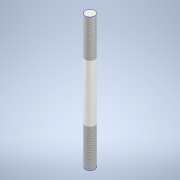
# Autodesk Inventor part: M5_60_shaft
Saved by Autodesk Inventor 2020.3 (Build 243373000, 373)
## iProperties
Created: 2021-03-23
Part Number: M5_60_shaft
Material: Aluminum 6061
Document SubType Name: Modeling
Designer: patry
Density: 2.7 g/cm^3
Appearance: Aluminum - Flat
Mass: 4.09976 g
Surface Area: 13.0959 cm^2
Volume: 1.51843 cm^3
Author: patry
Autodesk Inventor part; units mm, degrees
ref_plane "YZ Plane" through (0, 0, 0) normal (1, 0, 0) x (0, 1, 0)
ref_plane "XZ Plane" through (0, 0, 0) normal (0, 1, 0) x (-1, 0, 0)
ref_plane "XY Plane" through (0, 0, 0) normal (0, 0, 1) x (1, 0, 0)
sketch "Szkic1" plane through (0, 0, 0) normal (0, 1, 0) x (-1, 0, 0)
  circle A0 centre (0, 0) radius 4.25
  line L0 (1.1547, 2) -> (2.3094, 0)
  line L1 (2.3094, 0) -> (1.1547, -2)
  line L2 (1.1547, -2) -> (-1.1547, -2)
  line L3 (-1.1547, -2) -> (-2.3094, 0)
  line L4 (-2.3094, 0) -> (-1.1547, 2)
  line L5 (-1.1547, 2) -> (1.1547, 2)
  circle A1 centre (0, 0) radius 2.5
  dimension "d0" = 8.5
  dimension "d1" = 4
  dimension "d2" = 5
  constraints: 12 end point, 3 coincident, 2 centre point, 13 other
  measures "d0" diameter of A0
  measures "d1" distance between parallel lines of L2 L5
  measures "d2" diameter of A1
extrude "Wyciągnięcie proste4" add sketch "Szkic1" along normal blind 70 contours L0 L1 L2 L3 L4 L5 | A1
thread "Gwint2" size "M5x0.8" class "6g" standard "ANSI Metric M Profile" length 20
thread "Gwint3" size "M5x0.8" class "6g" standard "ANSI Metric M Profile" length 20
